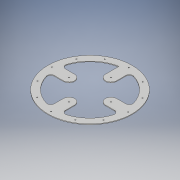
# Autodesk Inventor part: shell top bracket
Saved by Autodesk Inventor 2019 (Build 230136000, 136)
## iProperties
Created: 2019-02-10
Part Number: shell top bracket
Material: Generic
Document SubType Name: Modeling
Designer: mashimaro
Density: 1 g/cm^3
Appearance: Default
Author: mashimaro
Autodesk Inventor part; units mm, degrees
ref_plane "YZ Plane" through (0, 0, 0) normal (1, 0, 0) x (0, 1, 0)
ref_plane "XZ Plane" through (0, 0, 0) normal (0, 1, 0) x (-1, 0, 0)
ref_plane "XY Plane" through (0, 0, 0) normal (0, 0, 1) x (1, 0, 0)
sketch "Sketch1" plane through (0, 0, 0) normal (0, 1, 0) x (-1, 0, 0)
  circle A0 centre (60, 0) radius 1.5
  circle A1 centre (0, -60) radius 1.5
  circle A2 centre (-60, 0) radius 1.5
  circle A3 centre (0, 60) radius 1.5
  arc A4 (60, 16) -> (60, -16) centre (60, 0) ccw
  arc A5 (16, -60) -> (-16, -60) centre (0, -60) ccw
  arc A6 (-60, -16) -> (-60, 16) centre (-60, 0) ccw
  arc A7 (-16, 60) -> (16, 60) centre (0, 60) ccw
  circle A8 centre (0, 0) radius 120
  line L0 (16, 60) -> (16, 86.1626)
  line L1 (-16, 60) -> (-16, 86.1626)
  line L2 (-60, 16) -> (-86.1626, 16)
  line L3 (-60, -16) -> (-86.1626, -16)
  line L4 (-16, -60) -> (-16, -86.1626)
  line L5 (16, -60) -> (16, -98.7117)
  line L6 (60, 16) -> (86.1626, 16)
  line L7 (60, -16) -> (86.1626, -16)
  arc A9 (-28.8889, 95.7363) -> (-95.7363, 28.8889) centre (0, 0) ccw
  arc A10 (-95.7363, -28.8889) -> (-28.8889, -95.7363) centre (0, 0) ccw
  arc A11 (16, -98.7117) -> (95.7363, -28.8889) centre (0, 0) ccw
  arc A12 (95.7363, 28.8889) -> (28.8889, 95.7363) centre (0, 0) ccw
  arc A13 (28.8889, 95.7363) -> (16, 86.1626) centre (26, 86.1626) ccw
  arc A14 (86.1626, 16) -> (95.7363, 28.8889) centre (86.1626, 26) ccw
  arc A15 (95.7363, -28.8889) -> (86.1626, -16) centre (86.1626, -26) ccw
  arc A16 (-28.8889, -95.7363) -> (-16, -86.1626) centre (-26, -86.1626) ccw
  arc A17 (-86.1626, -16) -> (-95.7363, -28.8889) centre (-86.1626, -26) ccw
  arc A18 (-95.7363, 28.8889) -> (-86.1626, 16) centre (-86.1626, 26) ccw
  arc A19 (-16, 86.1626) -> (-28.8889, 95.7363) centre (-26, 86.1626) ccw
  line L8 (0, 0) -> (110, 0) construction
  circle A20 centre (95.8524, 53.966) radius 1.5
  circle A21 centre (56.0276, 94.6621) radius 1.5
  circle A22 centre (1.1903, 109.9936) radius 1.5
  circle A23 centre (-53.966, 95.8524) radius 1.5
  circle A24 centre (-94.6621, 56.0276) radius 1.5
  circle A25 centre (-109.9936, 1.1903) radius 1.5
  circle A26 centre (-95.8524, -53.966) radius 1.5
  circle A27 centre (-56.0276, -94.6621) radius 1.5
  circle A28 centre (-1.1903, -109.9936) radius 1.5
  circle A29 centre (53.966, -95.8524) radius 1.5
  circle A30 centre (94.6621, -56.0276) radius 1.5
  circle A31 centre (109.9936, -1.1903) radius 1.5
  point P0 (16, 98.7117)
  point P1 (-16, 98.7117)
  point P2 (-98.7117, 16)
  point P3 (-98.7117, -16)
  point P4 (-16, -98.7117)
  point P5 (98.7117, 16)
  point P6 (98.7117, -16)
  dimension "d1" = 3
  dimension "d2" = 3
  dimension "d3" = 3
  dimension "d4" = 3
  dimension "d5" = 32
  dimension "d6" = 32
  dimension "d7" = 32
  dimension "d8" = 32
  dimension "d14" = 10
  dimension "d17" = 3
  dimension "d20" = 360
  constraints: 37 point on circle, 32 centre point, 18 end point, 18 tangent, 9 point on line, 6 equal radius, 5 coincident, 2 horizontal, 2 parallel, 1 perpendicular, 1 vertical, 25 other
  measures "d1" diameter of A0
  measures "d2" diameter of A1
  measures "d3" diameter of A2
  measures "d4" diameter of A3
  measures "d5" diameter of A4
  measures "d6" diameter of A5
  measures "d7" diameter of A6
  measures "d8" diameter of A7
  measures "d14" radius of A13
  measures "d17" diameter of A20
extrude "Extrusion1" add sketch "Sketch1" along normal blind 2
body "Solid1"
